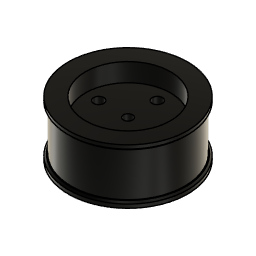
Back Wheel No Tire v6 (Autodesk Fusion 360 design; units mm, degrees)
Autodesk Fusion 360 part; units mm, degrees
note: some values were not read from the file. Set by a fixed rule: which sketch regions a step uses.
sketch "Main" plane through (0, 0, 0) normal (0, 0, 1) x (1, 0, 0)
  circle A0 centre (0, 0) radius 16.25
  dimension "d4" = 32.5
  constraint coincident A0.centre origin
  measures "d4" diameter of A0
extrude "Extrude2" add sketch "Main" along normal blind 15
sketch "Internal pocket" plane through (0, 0, 15) normal (0, 0, 1) x (-1, 0, 0)
  circle A0 centre (0, 0) radius 16.25
  circle A1 centre (0, 0) radius 11.6
  dimension "d49" = 23.2
  constraint coincident A0.centre A1.centre
  measures "d49" diameter of A1
sketch "External pocket" plane through (0, 0, 0) normal (0, 0, -1) x (1, 0, 0)
  circle A0 centre (0, 0) radius 11.25
  circle A1 centre (0, 0) radius 16.25
  dimension "d21" = 22.5
  constraint coincident A0.centre A1.centre
  measures "d21" diameter of A0
extrude "Extrude6" cut sketch "External pocket" against normal blind 5 contours A0
fillet "Fillet2" radius 2 1 edges at (-10.4887, -4.0682, 0)
sketch "Grooves" plane through (0, 0, 0) normal (1, 0, 0) x (0, 1, 0)
  line L0 (16.25, 0) -> (16.25, 15)
  line L1 (-16.25, 0) -> (-16.25, 15)
  line L2 (-1, 15) -> (-1, 0)
  line L3 (1, 15) -> (1, 0)
  line L4 (1, 15) -> (-1, 15)
  line L5 (1, 0) -> (-1, 0)
  line L6 (0, 0) -> (-16.25, 0)
  line L7 (16.25, 0) -> (0, 0)
  line L8 (0, 15) -> (-16.25, 15)
  line L9 (16.25, 15) -> (0, 15)
  dimension "d40" = 2
  dimension "d64" = 1
  constraint coincident L2.start L9
  constraint coincident L3.start L9
  constraint vertical L2
  constraint vertical L3
  constraint coincident L2.end L5.end
  constraint coincident L3.end L5.start
  constraint horizontal L5
  constraint coincident L6.start L5
  measures "d40" distance of L2.end L3.end
  measures "d64" distance of L2.start L8.start
extrude "Extrude10" cut sketch "Internal pocket" against normal blind 5 contours A1
sketch "Flange Holes" plane through (0, 0, 10) normal (0, 0, 1) x (-1, 0, 0)
  circle A0 centre (0, 0) radius 11.6
  circle A1 centre (8, 0) radius 1.4
  circle A2 centre (0, 8) radius 1.4
  circle A3 centre (-8, 0) radius 1.4
  circle A4 centre (0, -8) radius 1.4
  circle A5 centre (0, 0) radius 1.25
  dimension "d52" = 2.8
  dimension "d53" = 8
  dimension "d55" = 360
  dimension "d57" = 2.5
  constraint horizontal A0.centre A1.centre
  constraint concentric A0 A5
  measures "d52" diameter of A1
  measures "d53" distance of A0.centre A1.centre
  measures "d57" diameter of A5
extrude "Extrude11" cut sketch "Flange Holes" against normal through all contours A1 | A2 | A3 | A4
extrude "Extrude12" cut sketch "Flange Holes" against normal blind 2 contours A5
sketch "Tire pocket" plane through (0, 0, 15) normal (0, 0, 1) x (-1, 0, 0)
  circle A0 centre (0, 0) radius 11.6
  circle A1 centre (0, 0) radius 16.25
  circle A2 centre (0, 0) radius 15.5
  dimension "d65" = 31
  constraint coincident A0.centre A1.centre
  measures "d65" diameter of A2
extrude "Extrude13" cut sketch "Tire pocket" against normal blind 12 from surface at -1.5 contours A1
chamfer "Chamfer1" distance 0.5 angle 45 2 edges at (-15.1503, 5.8763, 1.5) (-15.1503, -5.8763, 13.5)
